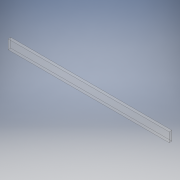
# Autodesk Inventor part: Front
Saved by Autodesk Inventor 2017 (Build 210142000, 142)
## iProperties
Created: 2017-04-17
Part Number: Front
Material: Generic
Document SubType Name: Modeling
Designer: jeffkub
Density: 1 g/cm^3
Appearance: Polycarbonate - Clear
Author: jeffkub
Autodesk Inventor part; units mm, degrees
ref_plane "YZ Plane" through (0, 0, 0) normal (1, 0, 0) x (0, 1, 0)
ref_plane "XZ Plane" through (0, 0, 0) normal (0, 1, 0) x (-1, 0, 0)
ref_plane "XY Plane" through (0, 0, 0) normal (0, 0, 1) x (1, 0, 0)
sketch "Sketch1" plane through (0, 0, 0) normal (0, 0, 1) x (1, 0, 0)
  line L0 (89.1, -5.2) -> (-89.1, -5.2)
  line L1 (-89.1, -5.2) -> (-89.1, 5.2)
  line L2 (-89.1, 5.2) -> (89.1, 5.2)
  line L3 (89.1, 5.2) -> (89.1, -5.2)
  line L4 (89.1, -5.2) -> (-89.1, 5.2) construction
  line L5 (-89.1, -5.2) -> (89.1, 5.2) construction
  point P0 (0, 0)
  dimension "d0" = 10.4
  dimension "d1" = 178.2
  constraints: 12 end point, 2 midpoint, 2 parallel, 1 horizontal, 1 perpendicular
  measures "d0" distance of L2.end L0.start
  measures "d1" distance of L1.end L2.end
extrude "Extrusion1" add sketch "Sketch1" along normal blind 3
body "Solid1"
